Autodesk Fusion 360 part; units mm, degrees
(part 2 of 2)
extrude "Extrude1" add sketch "Sketch1" along normal blind 3 contours A0 L0 L1 A3 L2 L3 L4 L5 L6 L7 L8 A8 L9 L10 L11 L12 L13 L15 L16 L18 L19 L20 L21 A13 L22 A782 A783 A784 A785 A786 A787 A788 A789 L23 L24 L25 A791 A792 A793 A794 L26 L27 L28 A796 A797 A798 A799 | A14 A18 A26 A29 A66 A73 A87 A88 A115 A123 A124 A130 A134 A154 A174 A191 A250 A254 A306 A313 A323 A326 A328 A337 A338 A339 A340 A345 A347 A348 A364 A380 | A15 A20 A22 A27 A64 A65 A77 A83 A129 A131 A138 A159 A171 A176 A193 A200 A222 A226 A232 A234 A235 A245 A261 A277 A285 A289 A295 A310 A357 A376 A381 A385 | A16 A19 A24 A28 A68 A72 A105 A109 A121 A127 A136 A156 A158 A166 A184 A190 A247 A251 A255 A256 A263 A264 A276 A283 A293 A307 A314 A319 A320 A336 A359 A383 | A17 A21 A23 A25 A69 A86 A92 A102 A128 A133 A155 A167 A180 A182 A197 A202 A219 A220 A221 A227 A230 A241 A257 A260 A270 A279 A291 A369 A371 A386 A387 A394 | A30 A93 A126 A169 A267 A312 A316 A389 | A31 A84 A151 A163 A215 A290 A362 A395 | A32 A104 A157 A195 A233 A294 A365 A374 | A33 A82 A116 A147 A262 A288 A324 A325 | A34 A71 A120 A185 A259 A265 A309 A317 | A35 A90 A140 A173 A206 A210 A212 A213 | A36 A67 A118 A139 A207 A208 A297 A299 | A37 A108 A114 A122 A209 A211 A296 A300 | A38 A96 A150 A204 A266 A382 A384 A390 | A39 A97 A144 A179 A268 A287 A366 A373 | A40 A91 A145 A177 A282 A358 A372 A379 | A41 A70 A132 A188 A253 A305 A311 A333 | A42 A89 A189 A196 A273 A274 A286 A363 | A43 A79 A153 A199 A301 A302 A341 A342 | A44 A95 A152 A201 A303 A304 A331 A349 | A45 A80 A141 A175 A284 A308 A315 A344 | A46 A103 A119 A178 A223 A321 A329 A355 | A47 A106 A165 A203 A249 A281 A334 A346 | A48 A107 A162 A192 A236 A278 A327 A354 | A49 A78 A187 A198 A280 A332 A335 A367 | A50 A63 A117 A142 A318 A322 A330 A343 | A51 A81 A183 A186 A214 A217 A298 A353 | A52 A75 A135 A143 A224 A225 A231 A350 | A53 A76 A137 A146 A216 A239 A351 A352 | A54 A99 A110 A112 A246 A361 A377 A396 | A55 A101 A113 A168 A218 A237 A240 A388 | A56 A98 A111 A164 A229 A370 A392 A397 | A57 A94 A125 A205 A228 A244 A356 A391 | A58 A74 A148 A170 A242 A243 A252 A275 | A59 A85 A149 A161 A258 A269 A360 A375 | A60 A100 A181 A194 A272 A292 A368 A378 | A61 A62 A160 A172 A238 A248 A271 A393 | A398 A416 A419 A421 A569 A574 A645 A747 | A399 A409 A575 A644 A658 A661 A671 A775 | A400 A402 A404 A406 A418 A420 A426 A572 | A401 A403 A405 A411 A412 A423 A571 A776 | A407 A408 A422 A570 A573 A641 A646 A748 | A410 A414 A417 A750 A774 A777 A779 A781 | A413 A424 A567 A576 A640 A751 A752 A780 | A415 A425 A568 A649 A653 A749 A753 A778 | A427 A435 A437 A438 A551 A694 A721 A728 | A428 A431 A517 A519 A690 A692 A706 A731 | A429 A443 A445 A452 A542 A561 A718 A744 | A430 A434 A442 A447 A449 A451 A472 A508 A521 A525 A531 A540 A541 A545 A548 A550 A563 A566 A678 A681 A691 A696 A701 A703 A708 A712 A715 A720 A723 A724 A735 A743 | A432 A444 A446 A471 A480 A484 A489 A490 A493 A495 A511 A512 A515 A520 A530 A533 A579 A597 A598 A682 A683 A685 A693 A697 A707 A711 A716 A719 A729 A732 A733 A737 | A433 A440 A448 A677 A722 A734 A742 A746 | A436 A513 A534 A535 A537 A679 A686 A738 | A439 A441 A547 A553 A554 A555 A556 A560 | A450 A475 A498 A522 A689 A698 A709 A726 | A453 A454 A462 A465 A651 A659 A664 A673 | A455 A458 A464 A467 A470 A543 A549 A565 | A456 A457 A469 A656 A657 A663 A668 A669 | A459 A463 A466 A559 A643 A648 A660 A670 | A460 A544 A546 A552 A557 A558 A562 A564 | A461 A468 A652 A662 A666 A672 A674 A675 | A473 A476 A477 A485 A496 A497 A501 A503 A504 A518 A523 A527 A529 A532 A538 A582 A586 A588 A594 A599 A684 A688 A699 A700 A704 A705 A710 A713 A714 A727 A730 A745 | A474 A487 A502 A578 A589 A619 A631 A639 | A478 A486 A506 A516 A536 A581 A587 A601 | A479 A481 A483 A505 A577 A580 A627 A635 | A482 A491 A500 A526 A528 A583 A592 A600 | A488 A499 A584 A585 A590 A591 A595 A596 | A492 A507 A509 A510 A514 A524 A539 A687 | A494 A602 A603 A604 A605 A606 A607 A609 A610 A612 A613 A617 A618 A621 A622 A623 A624 A626 A629 A630 A633 A634 A636 A637 A638 A702 A758 A759 A761 A767 A769 A771 | A593 A608 A611 A616 A620 A628 A757 A772 | A614 A615 A632 A755 A756 A762 A763 A766 | A625 A754 A760 A764 A765 A768 A770 A773 | A642 A647 A650 A654 A655 A665 A667 A676 | A680 A695 A717 A725 A736 A739 A740 A741 | A790 | A795
sketch "Sketch2" plane through (0, 3, 0) normal (0, 1, 0) x (-1, 0, 0)
  circle A0 centre (-15, -105) radius 2.75
  circle A1 centre (-184, -165) radius 2.75
  circle A2 centre (-184, -135) radius 2.75
  circle A3 centre (-184, -105) radius 2.75
  circle A4 centre (-15, -15) radius 2.75
  circle A5 centre (-184, -45) radius 2.75
  circle A6 centre (-15, -135) radius 2.75
  circle A7 centre (-15, -165) radius 2.75
  circle A8 centre (-15, -45) radius 2.75
  circle A9 centre (-184, -15) radius 2.75
  line L0 (-28, -115) -> (-5, -115)
  line L1 (0, -110) -> (0, -70)
  line L2 (-5, -65) -> (-28, -65)
  line L3 (-31, -62) -> (-31, -58)
  line L4 (-28, -55) -> (-5, -55)
  line L5 (0, -50) -> (0, -10)
  arc A10 (0, -10) -> (-10, 0) centre (-10, -10) ccw
  line L6 (-10, 0) -> (-189, 0)
  arc A11 (-189, 0) -> (-199, -10) centre (-189, -10) ccw
  line L7 (-199, -10) -> (-199, -50)
  line L8 (-194, -55) -> (-171, -55)
  line L9 (-168, -58) -> (-168, -62)
  line L10 (-171, -65) -> (-194, -65)
  line L11 (-194, -115) -> (-171, -115)
  line L12 (-168, -118) -> (-168, -122)
  line L13 (-171, -125) -> (-194, -125)
  line L14 (-199, -130) -> (-199, -170)
  arc A12 (-199, -170) -> (-189, -180) centre (-189, -170) ccw
  line L15 (-189, -180) -> (-10, -180)
  arc A13 (-10, -180) -> (0, -170) centre (-10, -170) ccw
  line L16 (0, -170) -> (0, -130)
  line L17 (-5, -125) -> (-28, -125)
  line L18 (-31, -122) -> (-31, -118)
  circle A14 centre (-50, -40) radius 10
  circle A15 centre (-50, -140) radius 10
  circle A16 centre (-110, -140) radius 10
  circle A17 centre (-110, -90) radius 12.5
  circle A18 centre (-110, -40) radius 10
  circle A19 centre (-160, -90) radius 1.75
  circle A20 centre (-150, -90) radius 1.75
  circle A21 centre (-140, -90) radius 1.75
  circle A22 centre (-130, -90) radius 1.75
  circle A23 centre (-90, -90) radius 1.75
  circle A24 centre (-80, -90) radius 1.75
  circle A25 centre (-70, -90) radius 1.75
  circle A26 centre (-60, -90) radius 1.75
  circle A27 centre (-50, -90) radius 1.75
  line L19 (-10, 0) -> (-189, 0)
  line L20 (0, -60) -> (0, -30)
  line L21 (0, -142) -> (0, -128.1084)
  line L22 (-10, -180) -> (-189, -180)
  circle A28 centre (-99.8, -157.5) radius 1.75
  circle A29 centre (-122.8, -157.5) radius 1.75
  circle A30 centre (-121.5, -122.5) radius 1.75
  circle A31 centre (-98.5, -122.5) radius 1.75
  arc A32 (-168, -58) -> (-171, -55) centre (-171, -58) ccw
  arc A33 (-171, -65) -> (-168, -62) centre (-171, -62) ccw
  arc A34 (-168, -118) -> (-171, -115) centre (-171, -118) ccw
  arc A35 (-171, -125) -> (-168, -122) centre (-171, -122) ccw
  arc A36 (-31, -122) -> (-28, -125) centre (-28, -122) ccw
  arc A37 (-28, -115) -> (-31, -118) centre (-28, -118) ccw
  arc A38 (-31, -62) -> (-28, -65) centre (-28, -62) ccw
  arc A39 (-28, -55) -> (-31, -58) centre (-28, -58) ccw
  circle A40 centre (-98.5, -57.5) radius 1.75
  circle A41 centre (-120.2, -22.5) radius 1.75
  circle A42 centre (-97.2, -22.5) radius 1.75
  circle A43 centre (-121.5, -57.5) radius 1.75
  arc A44 (-199, -50) -> (-194, -55) centre (-194, -50) ccw
  arc A45 (-194, -65) -> (-199, -70) centre (-194, -70) ccw
  line L23 (-199, -70) -> (-199, -110)
  arc A46 (-199, -110) -> (-194, -115) centre (-194, -110) ccw
  arc A47 (-194, -125) -> (-199, -130) centre (-194, -130) ccw
  arc A48 (0, -130) -> (-5, -125) centre (-5, -130) ccw
  arc A49 (-5, -115) -> (0, -110) centre (-5, -110) ccw
  arc A50 (0, -70) -> (-5, -65) centre (-5, -70) ccw
  arc A51 (-5, -55) -> (0, -50) centre (-5, -50) ccw
  point P0 (-63, -24)
  point P1 (-63, -24)
  point P2 (-64.3, -156)
  point P3 (-63, -121.74)
  dimension "d468" = 20
  dimension "d472" = 20
  dimension "d477" = 20
  dimension "d478" = 25
  dimension "d479" = 20
  dimension "d480" = 50
  dimension "d483" = 3.5
  dimension "d486" = 30
  dimension "d487" = 0
  dimension "d488" = 3.5
  dimension "d491" = 40
  dimension "d492" = 0
  dimension "d508" = 50
  dimension "d509" = 50
  dimension "d513" = 40
  dimension "d514" = 40
  dimension "d515" = 3.5
  dimension "d516" = 3.5
  dimension "d517" = 3.5
  dimension "d518" = 3.5
  dimension "d519" = 23
  dimension "d520" = 23
  dimension "d521" = 35
  dimension "d522" = 35
  dimension "d556" = 3.5
  dimension "d557" = 3.5
  dimension "d558" = 3.5
  dimension "d559" = 3.5
  dimension "d560" = 23
  dimension "d561" = 23
  dimension "d562" = 35
  dimension "d563" = 35
  dimension "d564" = 11.5
  dimension "d565" = 17.5
  dimension "d567" = 11.5
  dimension "d568" = 17.5
  measures "d468" diameter of A14
  measures "d472" diameter of A15
  measures "d477" diameter of A16
  measures "d478" diameter of A17
  measures "d479" diameter of A18
  measures "d480" distance of A17.centre A18.centre
  measures "d483" diameter of A19
  measures "d488" diameter of A23
  measures "d508" distance of A14.centre L20
  measures "d509" distance of A15.centre L21
  measures "d513" distance of A14.centre L19
  measures "d514" distance of A15.centre L22
  measures "d515" diameter of A28
  measures "d516" diameter of A29
  measures "d517" diameter of A31
  measures "d518" diameter of A30
  measures "d519" distance of A28.centre A29.centre
  measures "d520" horizontal distance of A30.centre A31.centre
  measures "d521" vertical distance of A29.centre A30.centre
  measures "d522" vertical distance of A28.centre A31.centre
  measures "d556" diameter of A40
  measures "d557" diameter of A43
  measures "d558" diameter of A42
  measures "d559" diameter of A41
  measures "d560" distance of A40.centre A43.centre
  measures "d561" horizontal distance of A42.centre A41.centre
  measures "d562" vertical distance of A43.centre A41.centre
  measures "d563" vertical distance of A40.centre A42.centre
  measures "d564" horizontal distance of A16.centre A30.centre
  measures "d565" vertical distance of A16.centre A28.centre
  measures "d567" horizontal distance of A18.centre A43.centre
  measures "d568" vertical distance of A18.centre A43.centre
extrude "Extrude2" cut sketch "Sketch2" against normal blind 3 contours A14
extrude "Extrude4" cut sketch "Sketch2" against normal blind 3 contours A15
extrude "Extrude5" cut sketch "Sketch2" against normal blind 3 contours A16 | A17 | A18
extrude "Extrude6" cut sketch "Sketch2" against normal blind 3 contours A19 | A20 | A21 | A22 | A23 | A24 | A25 | A26 | A27
extrude "Extrude7" add sketch "Sketch2" against normal blind 3 contours A14
extrude "Extrude8" add sketch "Sketch2" against normal blind 3 contours A15
extrude "Extrude9" cut sketch "Sketch2" against normal blind 3 contours A14 | A15 | A28 | A29 | A30 | A31
extrude "Extrude10" cut sketch "Sketch1" along normal blind 3 contours A14 A18 A26 A29 A66 A73 A87 A88 A115 A123 A124 A130 A134 A154 A174 A191 A250 A254 A306 A313 A323 A326 A328 A337 A338 A339 A340 A345 A347 A348 A364 A380 | A15 A20 A22 A27 A64 A65 A77 A83 A129 A131 A138 A159 A171 A176 A193 A200 A222 A226 A232 A234 A235 A245 A261 A277 A285 A289 A295 A310 A357 A376 A381 A385 | A16 A19 A24 A28 A68 A72 A105 A109 A121 A127 A136 A156 A158 A166 A184 A190 A247 A251 A255 A256 A263 A264 A276 A283 A293 A307 A314 A319 A320 A336 A359 A383 | A17 A21 A23 A25 A69 A86 A92 A102 A128 A133 A155 A167 A180 A182 A197 A202 A219 A220 A221 A227 A230 A241 A257 A260 A270 A279 A291 A369 A371 A386 A387 A394 | A30 A93 A126 A169 A267 A312 A316 A389 | A31 A84 A151 A163 A215 A290 A362 A395 | A32 A104 A157 A195 A233 A294 A365 A374 | A33 A82 A116 A147 A262 A288 A324 A325 | A34 A71 A120 A185 A259 A265 A309 A317 | A35 A90 A140 A173 A206 A210 A212 A213 | A36 A67 A118 A139 A207 A208 A297 A299 | A37 A108 A114 A122 A209 A211 A296 A300 | A38 A96 A150 A204 A266 A382 A384 A390 | A39 A97 A144 A179 A268 A287 A366 A373 | A40 A91 A145 A177 A282 A358 A372 A379 | A41 A70 A132 A188 A253 A305 A311 A333 | A42 A89 A189 A196 A273 A274 A286 A363 | A43 A79 A153 A199 A301 A302 A341 A342 | A44 A95 A152 A201 A303 A304 A331 A349 | A45 A80 A141 A175 A284 A308 A315 A344 | A46 A103 A119 A178 A223 A321 A329 A355 | A47 A106 A165 A203 A249 A281 A334 A346 | A48 A107 A162 A192 A236 A278 A327 A354 | A49 A78 A187 A198 A280 A332 A335 A367 | A50 A63 A117 A142 A318 A322 A330 A343 | A51 A81 A183 A186 A214 A217 A298 A353 | A52 A75 A135 A143 A224 A225 A231 A350 | A53 A76 A137 A146 A216 A239 A351 A352 | A54 A99 A110 A112 A246 A361 A377 A396 | A55 A101 A113 A168 A218 A237 A240 A388 | A56 A98 A111 A164 A229 A370 A392 A397 | A57 A94 A125 A205 A228 A244 A356 A391 | A58 A74 A148 A170 A242 A243 A252 A275 | A59 A85 A149 A161 A258 A269 A360 A375 | A60 A100 A181 A194 A272 A292 A368 A378 | A61 A62 A160 A172 A238 A248 A271 A393 | A398 A416 A419 A421 A569 A574 A645 A747 | A399 A409 A575 A644 A658 A661 A671 A775 | A400 A402 A404 A406 A418 A420 A426 A572 | A401 A403 A405 A411 A412 A423 A571 A776 | A407 A408 A422 A570 A573 A641 A646 A748 | A410 A414 A417 A750 A774 A777 A779 A781 | A413 A424 A567 A576 A640 A751 A752 A780 | A415 A425 A568 A649 A653 A749 A753 A778 | A427 A435 A437 A438 A551 A694 A721 A728 | A428 A431 A517 A519 A690 A692 A706 A731 | A429 A443 A445 A452 A542 A561 A718 A744 | A430 A434 A442 A447 A449 A451 A472 A508 A521 A525 A531 A540 A541 A545 A548 A550 A563 A566 A678 A681 A691 A696 A701 A703 A708 A712 A715 A720 A723 A724 A735 A743 | A432 A444 A446 A471 A480 A484 A489 A490 A493 A495 A511 A512 A515 A520 A530 A533 A579 A597 A598 A682 A683 A685 A693 A697 A707 A711 A716 A719 A729 A732 A733 A737 | A433 A440 A448 A677 A722 A734 A742 A746 | A436 A513 A534 A535 A537 A679 A686 A738 | A439 A441 A547 A553 A554 A555 A556 A560 | A450 A475 A498 A522 A689 A698 A709 A726 | A453 A454 A462 A465 A651 A659 A664 A673 | A455 A458 A464 A467 A470 A543 A549 A565 | A456 A457 A469 A656 A657 A663 A668 A669 | A459 A463 A466 A559 A643 A648 A660 A670 | A460 A544 A546 A552 A557 A558 A562 A564 | A461 A468 A652 A662 A666 A672 A674 A675 | A473 A476 A477 A485 A496 A497 A501 A503 A504 A518 A523 A527 A529 A532 A538 A582 A586 A588 A594 A599 A684 A688 A699 A700 A704 A705 A710 A713 A714 A727 A730 A745 | A474 A487 A502 A578 A589 A619 A631 A639 | A478 A486 A506 A516 A536 A581 A587 A601 | A479 A481 A483 A505 A577 A580 A627 A635 | A482 A491 A500 A526 A528 A583 A592 A600 | A488 A499 A584 A585 A590 A591 A595 A596 | A492 A507 A509 A510 A514 A524 A539 A687 | A494 A602 A603 A604 A605 A606 A607 A609 A610 A612 A613 A617 A618 A621 A622 A623 A624 A626 A629 A630 A633 A634 A636 A637 A638 A702 A758 A759 A761 A767 A769 A771 | A593 A608 A611 A616 A620 A628 A757 A772 | A614 A615 A632 A755 A756 A762 A763 A766 | A625 A754 A760 A764 A765 A768 A770 A773 | A642 A647 A650 A654 A655 A665 A667 A676 | A680 A695 A717 A725 A736 A739 A740 A741
sketch "Sketch3" plane through (99.5, 0, -90) normal (0, 1, 0) x (1, 0, 0)
  line L0 (68.5, 90) -> (73.5, 90)
  line L1 (73.5, 90) -> (73.5, -90)
  line L2 (73.5, -90) -> (68.5, -90)
  line L3 (68.5, -90) -> (68.5, 90)
  line L4 (99.5, 60) -> (99.5, 25)
  line L5 (-68.5, 90) -> (-73.5, 90)
  line L6 (-73.5, 90) -> (-73.5, -90)
  line L7 (-73.5, -90) -> (-68.5, -90)
  line L8 (-68.5, -90) -> (-68.5, 90)
  line L9 (-99.5, 60) -> (-99.5, 22)
  dimension "d531" = 5
  dimension "d532" = 31
  dimension "d533" = 5
  dimension "d534" = 31
  constraint horizontal L0
  constraint vertical L1
  constraint horizontal L2
  constraint vertical L3
  constraint horizontal L5
  constraint vertical L6
  constraint horizontal L7
  constraint vertical L8
  measures "d531" distance of L1 L3
  measures "d532" distance of L3 L4
  measures "d533" distance of L6 L8
  measures "d534" distance of L8 L9
extrude "Extrude11" cut sketch "Sketch3" along normal blind 2
extrude "Extrude12" cut sketch "Sketch2" against normal blind 3 contours A28 | A29 | A30 | A31 | A40 | A41 | A42 | A43
extrude "Extrude13" cut sketch "Sketch1" along normal blind 3 contours A790 | A795
extrude "Extrude14" add 1 faces at (27.4102, 3, -90) along direction (0, 1, 0) blind 1
extrude "Extrude3" [suppressed]
